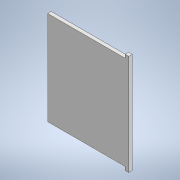
# Autodesk Inventor part: top lid
Saved by Autodesk Inventor 2020 (Build 240168000, 168)
## iProperties
Created: 2022-02-16
Part Number: top lid
Material: Generic
Document SubType Name: Modeling
Designer: rwte
Density: 1 g/cm^3
Appearance: Default
Author: rwte
Autodesk Inventor part; units mm, degrees
ref_plane "YZ Plane" through (0, 0, 0) normal (1, 0, 0) x (0, 1, 0)
ref_plane "XZ Plane" through (0, 0, 0) normal (0, 1, 0) x (-1, 0, 0)
ref_plane "XY Plane" through (0, 0, 0) normal (0, 0, 1) x (1, 0, 0)
sketch "Sketch1" plane through (0, 0, 0) normal (0, 0, 1) x (1, 0, 0)
  line L0 (-35, -40.5) -> (-35, 40.5)
  line L1 (-35, 40.5) -> (35, 40.5)
  line L2 (35, 40.5) -> (35, -40.5)
  line L3 (35, -40.5) -> (-35, -40.5)
  line L4 (-35, -40.5) -> (35, 40.5) construction
  line L5 (-35, 40.5) -> (35, -40.5) construction
  line L6 (35, -40.5) -> (32, -40.5)
  line L7 (32, -40.5) -> (32, -43.5)
  line L8 (32, -43.5) -> (35, -43.5)
  line L9 (35, -43.5) -> (35, -40.5)
  line L10 (-49, 0) -> (49, 0) projected
  line L11 (32, 40.5) -> (32, 43.5)
  line L12 (32, 43.5) -> (35, 43.5)
  line L13 (35, 43.5) -> (35, 40.5)
  point P0 (0, 0)
  dimension "d0" = 70
  dimension "d1" = 81
  dimension "d4" = 3
  dimension "d5" = 3
  constraints: 26 end point, 4 parallel, 3 symmetric about line, 2 midpoint, 2 perpendicular, 1 horizontal, 1 vertical
  measures "d0" distance of L2.end L0.start
  measures "d1" distance of L1.end L2.end
  measures "d4" distance of L8.end L2.end
  measures "d5" distance of L7.end L8.end
extrude "Extrusion1" add sketch "Sketch1" along normal blind 3
equation "\"d4\" = d2"
equation "\"d5\" = d2"
equation "\"d2\" = 3"
body "Solid1"
